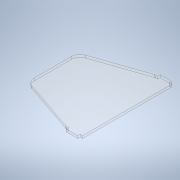
# Autodesk Inventor part: rearCover
Saved by Autodesk Inventor 2020 (Build 240168000, 168)
## iProperties
Created: 2020-03-02
Part Number: rearCover
Material: Polycarbonate, Clear
Document SubType Name: Modeling
Designer: n10208577
Density: 1.2 g/cm^3
Appearance: Polycarbonate - Clear
Author: n10208577
Autodesk Inventor part; units mm, degrees
ref_plane "YZ Plane" through (0, 0, 0) normal (1, 0, 0) x (0, 1, 0)
ref_plane "XZ Plane" through (0, 0, 0) normal (0, 1, 0) x (-1, 0, 0)
ref_plane "XY Plane" through (0, 0, 0) normal (0, 0, 1) x (1, 0, 0)
sketch "Sketch1" plane through (0, 0, 0) normal (0, 1, 0) x (-1, 0, 0)
  line L0 (9.0102, -12.8984) -> (9.0102, -15.8984)
  line L1 (9.0102, 95.1016) -> (9.0102, 98.1016)
  line L2 (9.0102, -15.8984) -> (-4.9898, -15.8984)
  line L3 (9.0102, 98.1016) -> (-4.9898, 98.1016)
  line L4 (-4.9898, 98.1016) -> (-4.9898, 95.1016)
  line L5 (-4.9898, 95.1016) -> (-7.9898, 95.1016)
  line L6 (-7.9898, 95.1016) -> (-7.9898, -12.8984)
  line L7 (-7.9898, -12.8984) -> (-4.9898, -12.8984)
  line L8 (-4.9898, -12.8984) -> (-4.9898, -15.8984)
  line L9 (9.0102, 95.1016) -> (11.1769, 95.1016)
  line L10 (11.1769, -12.8984) -> (9.0102, -12.8984)
  line L11 (82.0102, 18.2445) -> (82.0102, 63.9587)
  arc A0 (75.2535, 8.785) -> (82.0102, 18.2445) centre (72.0102, 18.2445) ccw
  arc A1 (82.0102, 63.9587) -> (75.2535, 73.4182) centre (72.0102, 63.9587) ccw
  line L12 (12.7985, -12.6281) -> (75.2535, 8.785)
  arc A2 (11.1769, -12.8984) -> (12.7985, -12.6281) centre (11.1769, -7.8984) ccw
  line L13 (12.7985, 94.8313) -> (75.2535, 73.4182)
  arc A3 (12.7985, 94.8313) -> (11.1769, 95.1016) centre (11.1769, 90.1016) ccw
  point P0 (0, 0)
  constraints: 28 end point, 8 point on circle, 4 centre point
extrude "Extrusion1" add sketch "Sketch1" along normal blind 3
body "Solid1"
